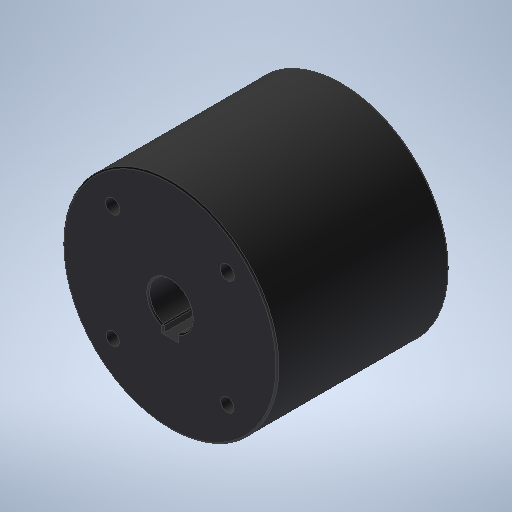
# Autodesk Inventor part: Flansch 3Ddruck
Saved by Autodesk Inventor 2025 (Build 290162000, 162)
## iProperties
Created: 2025-12-15
Part Number: Flansch 3Ddruck
Material: Generic
Document SubType Name: Modeling
Designer: ruven
Density: 1 g/cm^3
Appearance: Default
Author: ruven
Autodesk Inventor part; units mm, degrees
ref_plane "YZ Plane" through (0, 0, 0) normal (1, 0, 0) x (0, 1, 0)
ref_plane "XZ Plane" through (0, 0, 0) normal (0, 1, 0) x (-1, 0, 0)
ref_plane "XY Plane" through (0, 0, 0) normal (0, 0, 1) x (1, 0, 0)
sketch "Sketch1" plane through (0, 0, 0) normal (0, 1, 0) x (-1, 0, 0)
  circle A0 centre (-20, 20) radius 2.5
  circle A1 centre (-20.0115, -20) radius 2.3331
  circle A2 centre (20, 20) radius 2.5
  circle A3 centre (19.9885, -20) radius 2.3169
  circle A4 centre (0, -0.053) radius 37.5
  line L0 (2.55, -7.239) -> (2.55, -9.7779)
  line L1 (2.55, -9.7779) -> (-2.55, -9.789)
  line L2 (-2.55, -9.789) -> (-2.55, -7.239)
  line L3 (-2.55, -5.5721) -> (2.55, -9.7779) construction
  line L4 (2.55, -5.561) -> (-2.55, -9.789) construction
  line L5 (0, -0.053) -> (0, -12.2317) construction
  arc A5 (2.55, -7.239) -> (-2.55, -7.239) centre (0, -0.053) ccw
  point P0 (0, 0)
  point P1 (0, -7.675)
  point P2 (2.55, -8.5084)
  point P3 (-2.55, -8.514)
  dimension "d1" = 40
  dimension "d2" = 40
  dimension "d3" = 40
  dimension "d4" = 40
  dimension "d10" = 75
  dimension "d16" = 0
  dimension "d17" = 2.55
  dimension "d19" = 5.1
  dimension "d20" = 0
  dimension "d21" = 0
  dimension "d22" = 2.1084
  dimension "d24" = 7.625
  constraints: 12 end point, 6 centre point, 4 midpoint, 2 point on circle, 1 coincident, 1 parallel, 1 vertical
  measures "d1" distance of A3.centre A1.centre
  measures "d2" distance of A2.centre A3.centre
  measures "d3" distance of A0.centre A2.centre
  measures "d4" distance of A1.centre A0.centre
  measures "d10" diameter of A4
  measures "d16" horizontal distance of L5.start point (0, 0)
  measures "d17" horizontal distance of point (0, -7.675) point (2.55, -8.508)
  measures "d19" distance from line of point (-2.55, -8.514) L0
  measures "d20" distance from line of L5 point (0, -7.675)
  measures "d21" angle of L5 L0
  measures "d22" distance from line of point (0, -7.675) L1
  measures "d24" radius of A5
extrude "Extrusion1" add sketch "Sketch1" along normal blind 60
fillet "Fillet1" radius 0.5 4 edges at (37.5, 60, -0.053) (37.5, 0, -0.053) (0, 60, 7.572) (0, 0, 7.572)
fillet "Fillet2" radius 0.5 10 edges at (-2.55, 59.8545, -7.3953) (-2.55, 60, -8.7727) (-2.55, 0.1455, -7.3953) (-2.55, 0, -8.7727) (-2.55, 30, -7.239) (2.55, 59.8545, -7.3953) (2.55, 60, -8.7783) (2.55, 0.1455, -7.3953) (2.55, 0, -8.7783) (2.55, 30, -7.239)
body "Solid1"
